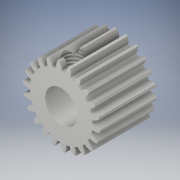
# Autodesk Inventor part: motor gear
Saved by Autodesk Inventor 2017 (Build 210142000, 142)
## iProperties
Created: 2016-06-11
Part Number: motor gear
Material: Generic
Document SubType Name: Modeling
Designer: Ben
Density: 1 g/cm^3
Appearance: Default
Author: Ben
Autodesk Inventor part; units mm, degrees
ref_plane "YZ Plane" through (0, 0, 0) normal (1, 0, 0) x (0, 1, 0)
ref_plane "XZ Plane" through (0, 0, 0) normal (0, 1, 0) x (-1, 0, 0)
ref_plane "XY Plane" through (0, 0, 0) normal (0, 0, 1) x (1, 0, 0)
sketch "Sketch2" plane through (0, 0, 0) normal (0, 0, 1) x (1, 0, 0)
  circle A0 centre (0, 0) radius 5.5
  line L0 (0, 0) -> (0, 27.6847) construction
  line L1 (-23.9445, 5.5) -> (24.9427, 5.5) construction
  line L2 (-20.499, -1.961) -> (20.499, 12.961) construction
  line L3 (0, 0) -> (-1.7677, 4.8566) construction
  arc A1 (-1.7677, 4.8566) -> (-2.8378, 4.3196) centre (0, 0) ccw
  line L4 (-2.8378, 4.3196) -> (-0.2626, 6.0113) construction
  arc A2 (-0.8008, 5.1059) -> (-1.7677, 4.8566) centre (0, 0) ccw
  line L5 (-0.8008, 5.1059) -> (0.0696, 5.2424) construction
  line L6 (0, 0) -> (-3.0155, 42.1618) construction
  circle A3 centre (0, 0) radius 5.1683 construction
  line L7 (0.0686, 5.1679) -> (0.0696, 5.2424) construction
  line L8 (0.0696, 5.2424) -> (0, 5.5) construction
  line L9 (0, 5.5) -> (-0.2626, 6.0113) construction
  spline S0 degree 3 poles (0.0686, 5.1679) (0.0696, 5.2424) (0, 5.5) (-0.2626, 6.0113) knots 1 1 1 1 2 2 2 2
  line L10 (0, 0) -> (-2.8378, 4.3196) construction
  line L11 (-0.8034, 5.1055) -> (-0.815, 5.1791) construction
  line L12 (-0.815, 5.1791) -> (-0.7827, 5.444) construction
  line L13 (-0.7827, 5.444) -> (-0.5955, 5.9875) construction
  spline S1 degree 3 poles (-0.8034, 5.1055) (-0.815, 5.1791) (-0.7827, 5.444) (-0.5955, 5.9875) knots 1 1 1 1 2 2 2 2
  line L14 (0.0686, 5.1679) -> (0.0686, 4.9179)
  line L15 (-0.8034, 5.1055) -> (-0.7678, 4.858)
  circle A4 centre (0, 0) radius 4.9183
  arc A5 (-0.2626, 6.0113) -> (-0.5955, 5.9875) centre (0, 0) ccw
  arc A6 (0.0686, 4.9179) -> (-0.7678, 4.858) centre (0, 0) ccw
  dimension "d0" = 11
  dimension "d1" = 20
  dimension "d6" = 1.8811
  dimension "d7" = 1
  dimension "d8" = 0.8811
  dimension "d9" = 4.091
  dimension "d61" = 1.2
  dimension "d62" = 3.0811
  dimension "d64" = 0.25
  constraints: 20 end point, 9 coincident, 8 point on circle, 5 centre point, 5 symmetric about line, 3 point on line, 3 tangent, 2 perpendicular, 2 vertical, 1 horizontal, 1 midpoint, 13 other
  measures "d0" diameter of A0
  measures "d1" angle of L1 L2
  measures "d6" distance of point (0, 5.5) L3.end
  measures "d8" distance of L5.start L5.end
  measures "d9" angle of L0 L6
  measures "d62" distance of L4.start L4.end
  measures "d64" distance of L7.start L14.end
sketch "Sketch4" plane through (0, 0, 0) normal (0, 0, 1) x (1, 0, 0)
  circle A0 centre (0, 0) radius 4.9183 projected
extrude "Extrusion1" add sketch "Sketch4" along normal blind 9
sketch "Sketch5" plane through (0, 0, 0) normal (0, 0, 1) x (1, 0, 0)
  spline S0 degree 3 poles (-0.8034, 5.1055) (-0.815, 5.1791) (-0.7827, 5.444) (-0.5955, 5.9875) knots 1 1 1 1 2 2 2 2 projected
  spline S1 degree 3 poles (0.0686, 5.1679) (0.0696, 5.2424) (0, 5.5) (-0.2626, 6.0113) knots 1 1 1 1 2 2 2 2 projected
  line L0 (0, 0) -> (-3.0155, 42.1618) construction
  arc A0 (-0.2626, 6.0113) -> (-0.5955, 5.9875) centre (0, 0) ccw projected
  line L1 (-0.8034, 5.1055) -> (-0.7678, 4.858) projected
  line L2 (0.0686, 5.1679) -> (0.0686, 4.9179) projected
  arc A1 (0.0686, 4.9179) -> (-0.7678, 4.858) centre (0, 0) ccw projected
extrude "Extrusion3" add sketch "Sketch5" along normal up to surface (9 mm away)
pattern_circular "Circular Pattern1" count 22 over 360 about axis through (0, 0, -10) along (0, 0, 1) of "Extrusion3"
sketch "Sketch24" plane through (0, 0, 0) normal (0, 0, 1) x (1, 0, 0)
  circle A0 centre (0, 0) radius 6
  circle A1 centre (0, 0) radius 12
  dimension "d121" = 12
  dimension "d122" = 24
  constraints: 2 centre point, 2 coincident
  measures "d121" diameter of A0
  measures "d122" diameter of A1
extrude "Extrusion12" cut sketch "Sketch24" along normal up to surface (9 mm away)
sketch "Sketch47" plane through (0, 0, 9) normal (0, 0, 1) x (1, 0, 0)
  circle A0 centre (0, 0) radius 2.5
  dimension "d183" = 5
  constraints: 1 centre point, 1 coincident
  measures "d183" diameter of A0
extrude "Extrusion19" cut sketch "Sketch47" against normal up to next
ref_plane "Work Plane16" through (0, 0, 0) normal (-0.0713392, 0.9974521, 0) x (-0.9974521, -0.0713392, 0)
sketch "Sketch48" plane through (0, 0, 0) normal (-0.0713392, 0.9974521, 0) x (-0.9974521, -0.0713392, 0)
  circle A0 centre (0, 6.8) radius 1.4
  line L0 (0, 0) -> (0, 5.7567) construction
  line L1 (-2.5, 9) -> (2.5, 9) projected
  dimension "d186" = 2.8
  dimension "d192" = 2.2
  constraints: 2 end point, 1 centre point, 1 point on line, 1 vertical
  measures "d186" diameter of A0
  measures "d192" distance from line of L1 A0.centre
extrude "Extrusion20" cut sketch "Sketch48" along normal up to next
thread "Thread1" size "M3x0.5" class "6H" standard "ANSI Metric M Profile" full length
ref_plane "Work Plane17" through (0, 0, 4.5) normal (0, 0, 1) x (1, 0, 0)
equation "\"d8\" = d6 - d7"
equation "\"m1\" = 0.5"
body "Solid1"
